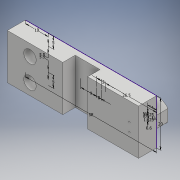
# Autodesk Inventor part: LDR_Holder
Saved by Autodesk Inventor 2017 (Build 210142000, 142)
## iProperties
Created: 2017-03-22
Part Number: LDR_Holder
Material: Generic
Document SubType Name: Modeling
Designer: willt
Density: 1 g/cm^3
Appearance: Default
Author: willt
Autodesk Inventor part; units mm, degrees
ref_plane "YZ Plane" through (0, 0, 0) normal (1, 0, 0) x (0, 1, 0)
ref_plane "XZ Plane" through (0, 0, 0) normal (0, 1, 0) x (-1, 0, 0)
ref_plane "XY Plane" through (0, 0, 0) normal (0, 0, 1) x (1, 0, 0)
sketch "Sketch1" plane through (0, 0, 0) normal (0, 1, 0) x (-1, 0, 0)
  line L0 (0, 0) -> (-58, 0)
  line L1 (-58, 0) -> (-58, -20)
  line L2 (-58, -20) -> (0, -20)
  line L3 (0, -20) -> (0, 0)
  line L4 (-58, -10) -> (-54, -10) construction
  arc A0 (-56, -11.8875) -> (-52, -11.8875) centre (-54, -10) ccw
  line L5 (-58, -10) -> (-56, -10) construction
  line L6 (-56, -10) -> (-56, -11.8875)
  line L7 (-56, -10) -> (-56, -8.1125)
  line L8 (-54, -10) -> (-52, -10) construction
  line L9 (-52, -10) -> (-52, -11.8875)
  line L10 (-52, -10) -> (-52, -8.1125)
  arc A1 (-52, -8.1125) -> (-56, -8.1125) centre (-54, -10) ccw
  arc A2 (-58, -12.5617) -> (-58, -7.4383) centre (-54, -10) ccw
  line L11 (0, 0) -> (-10, 0) construction
  line L12 (-10, 0) -> (-10, -5) construction
  line L13 (-10, -20) -> (-10, -15) construction
  circle A3 centre (-10, -5) radius 2.75
  circle A4 centre (-10, -15) radius 2.75
  line L14 (-54, -10) -> (-54, -11.925) construction
  line L15 (-54, -10) -> (-54, -8.075) construction
  circle A5 centre (-54, -8.075) radius 0.3
  circle A6 centre (-54, -11.925) radius 0.3
  line L16 (-58, -10) -> (-31.5, -10) construction
  line L17 (-33.5, -10) -> (-24.5, -10) construction
  line L18 (-35.5, -20) -> (-35.5, 0)
  line L19 (-24.5, -20) -> (-24.5, 0)
  line L20 (-31.5, -10) -> (-33.5, -10) construction
  line L21 (-33.5, -10) -> (-35.5, -10) construction
  line L22 (-24.5, 0) -> (-35.5, 0)
  line L23 (-35.5, 0) -> (-35.5, -20)
  line L24 (-35.5, -20) -> (-24.5, -20)
  line L25 (-24.5, -20) -> (-24.5, 0)
  dimension "d0" = 58
  dimension "d1" = 20
  dimension "d2" = 4
  dimension "d4" = 2
  dimension "d5" = 2
  dimension "d7" = 10
  dimension "d8" = 5
  dimension "d9" = 5
  dimension "d10" = 5.5
  dimension "d11" = 5.5
  dimension "d18" = 1.925
  dimension "d19" = 1.925
  dimension "d20" = 0.6
  dimension "d21" = 0.6
  dimension "d24" = 26.5
  dimension "d25" = 9
  dimension "d32" = 2
  dimension "d33" = 2
  constraints: 52 end point, 10 point on line, 7 centre point, 7 perpendicular, 7 point on circle, 5 coincident, 4 horizontal, 4 parallel, 3 vertical, 2 midpoint
  measures "d0" distance of L2.end L1.end
  measures "d1" distance of L1.end L0.end
  measures "d2" distance of L4.start L4.end
  measures "d4" distance of L4.start L5.end
  measures "d5" distance of L8.start L8.end
  measures "d7" distance of L0.start L11.end
  measures "d8" distance of L11.end L12.end
  measures "d9" distance of L13.start L13.end
  measures "d10" diameter of A3
  measures "d11" diameter of A4
  measures "d18" distance of L14.start L14.end
  measures "d19" distance of L14.start L15.end
  measures "d20" diameter of A5
  measures "d21" diameter of A6
  measures "d24" distance of L16.end L4.start
  measures "d25" distance of L17.start L17.end
  measures "d32" distance of L16.end L17.start
  measures "d33" distance of L17.start L21.end
extrude "Extrusion2" add sketch "Sketch1" against normal blind 8 contours A2 L1
extrude "Extrusion3" add sketch "Sketch1" along normal blind 5 contours A2 L1
extrude "Extrusion4" add sketch "Sketch1" against normal blind 8 contours L6 L7 A1 L10 L9 A0
extrude "Extrusion8" add sketch "Sketch1" against normal blind 8 contours L3 L2 L19 L0 | L18 L2 L1 A2 L0
extrude "Extrusion9" add sketch "Sketch1" against normal blind 2.5 contours L19 L2 L18 L0
body "Solid1"
